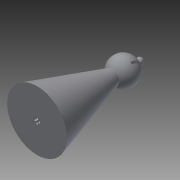
# Autodesk Inventor part: fou
Saved by Autodesk Inventor 2015 (Build 190159000, 159)
## iProperties
Created: 2015-02-16
Part Number: fou
Material: Générique
Document SubType Name: Modeling
Designer: informatique
Density: 1 g/cm^3
Appearance: Par défaut
Author: informatique
Autodesk Inventor part; units mm, degrees
ref_plane "YZ Plane" through (0, 0, 0) normal (1, 0, 0) x (0, 1, 0)
ref_plane "XZ Plane" through (0, 0, 0) normal (0, 1, 0) x (-1, 0, 0)
sketch "Esquisse1" plane through (0, 0, 0) normal (1, 0, 0) x (0, 1, 0)
  line L0 (0, 0) -> (0, -9)
  line L1 (0, 0) -> (30, 0)
  line L2 (22.6606, -2.2018) -> (0, -9)
  arc A0 (22.6606, -2.2018) -> (30, 0) centre (26, 0) ccw
  circle A1 centre (31, 0) radius 1
  line L3 (30, 0) -> (32, 0)
  dimension "d0" = 9
  dimension "d1" = 30
  dimension "d2" = 4
  dimension "d3" = 1
  constraints: 8 end point, 4 point on circle, 2 centre point, 2 horizontal, 1 point on line, 1 vertical
  measures "d0" distance of L0.start L0.end
  measures "d1" distance of L0.start L1.end
  measures "d2" distance of A0.centre L1.end
  measures "d3" distance of L1.end A1.centre
revolve "Révolution1" add sketch "Esquisse1" angle 360 about axis through (0, 0, 0) along (0, 1, 0) picked at (30.9598, -0.3309) contours L1 A0 L2 L0 | L3 A1
ref_plane "Plan de construction5" through (0, 31, 0) normal (0, -1, 0) x (1, 0, 0)
sketch "Esquisse2" plane through (0, 31, 0) normal (0, -1, 0) x (1, 0, 0)
  circle A0 centre (0, 0) radius 4 projected
  line L0 (2.1458, -5) -> (2.6458, -5)
  line L1 (2.6458, -5) -> (2.6458, 3)
  line L2 (2.6458, 3) -> (2.1458, 3)
  line L3 (2.1458, 3) -> (2.1458, -5)
  line L4 (2.1458, 3) -> (2.6458, 3)
  line L5 (2.6458, 3) -> (2.6458, 4.2715)
  line L6 (2.6458, 4.2715) -> (2.1458, 4.2715)
  line L7 (2.1458, 4.2715) -> (2.1458, 3)
  dimension "d12" = 5
  dimension "d13" = 8
  constraints: 16 end point, 4 parallel, 2 horizontal, 2 perpendicular, 2 other
  measures "d12" vertical distance of point (0, 0) L0.start
  measures "d13" distance of L0.end L1.end
extrude "Extrusion1" cut sketch "Esquisse2" along normal blind 5 contours L2 L7 A0 | L1 A0 L3 L2 | A0 L7 L6 L5 | L1 L0 L3 A0
sketch "Esquisse3" plane through (0, 0, 0) normal (0, -1, 0) x (1, 0, 0)
  line L0 (-0.3714, 0.9357) -> (0.3286, 0.9357)
  line L1 (0.3286, 0.9357) -> (0.3286, -0.9643)
  line L2 (0.3286, -0.9643) -> (-0.3714, -0.9643)
  line L3 (-0.3714, -0.9643) -> (-0.3714, 0.9357)
  line L4 (0.9286, 0.3357) -> (-0.9714, 0.3357)
  line L5 (-0.9714, 0.3357) -> (-0.9714, -0.3643)
  line L6 (-0.9714, -0.3643) -> (0.9286, -0.3643)
  line L7 (0.9286, -0.3643) -> (0.9286, 0.3357)
  point P0 (0, 0)
  point P1 (0, 0)
  dimension "d16" = 0.7
  dimension "d17" = 0.7
  dimension "d18" = 1.9
  dimension "d19" = 1.9
  dimension "d20" = 0.6
  dimension "d21" = 0.6
  constraints: 16 end point, 4 parallel, 2 horizontal, 2 perpendicular
  measures "d16" distance of L0.start L0.end
  measures "d17" distance of L6.end L4.start
  measures "d18" distance of L5.end L6.end
  measures "d19" distance of L2.end L0.start
  measures "d20" distance between parallel lines of L6 L2
  measures "d21" distance between parallel lines of L3 L5
extrude "Extrusion2" cut sketch "Esquisse3" against normal blind 10
